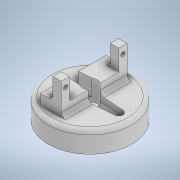
# Autodesk Inventor part: Part1
Saved by Autodesk Inventor 2020.2 (Build 242310000, 310)
## iProperties
Created: 2026-04-23
Part Number: Part1
Material: Generic
Document SubType Name: Modeling
Designer: explorer
Density: 1 g/cm^3
Appearance: Default
Author: explorer
Autodesk Inventor part; units mm, degrees
ref_plane "YZ Plane" through (0, 0, 0) normal (1, 0, 0) x (0, 1, 0)
ref_plane "XZ Plane" through (0, 0, 0) normal (0, 1, 0) x (-1, 0, 0)
ref_plane "XY Plane" through (0, 0, 0) normal (0, 0, 1) x (1, 0, 0)
sketch "Sketch1" plane through (0, 0, 0) normal (0, 1, 0) x (-1, 0, 0)
  circle A0 centre (0, 0) radius 20
  circle A1 centre (0, 0) radius 3.5
  dimension "d10" = 40
  dimension "d115" = 7
  constraints: 2 centre point, 2 coincident
  measures "d10" diameter of A0
  measures "d115" diameter of A1
extrude "Extrusion1" add sketch "Sketch1" along normal blind 10
sketch "Sketch3" plane through (0, 0, 0) normal (0, -1, 0) x (1, 0, 0)
  circle A0 centre (0, 0) radius 15
  dimension "d16" = 30
  constraints: 1 centre point, 1 coincident
  measures "d16" diameter of A0
extrude "Extrusion3" cut sketch "Sketch3" against normal blind 5
sketch "Sketch4" plane through (0, 10, 0) normal (0, 1, 0) x (1, 0, 0)
  circle A0 centre (-15.75, 0) radius 2 construction
  line L0 (0, 0) -> (-15.75, 0) construction
  arc A1 (-13.75, 2) -> (-13.75, -2) centre (-13.75, 0) ccw
  line L1 (-13.75, 0) -> (-13.75, 2) construction
  line L2 (-13.75, 0) -> (-11.75, 0) construction
  line L3 (-13.75, 0) -> (-13.75, -2) construction
  circle A2 centre (0, 0) radius 3.5 construction
  circle A3 centre (0, 0) radius 3 construction
  line L4 (0, 28) -> (0, -28) construction
  line L5 (-28, 0) -> (28, 0) construction
  line L6 (-13.75, 2) -> (0, 3)
  line L7 (-13.75, -2) -> (0, -3)
  arc A4 (13.75, -2) -> (13.75, 2) centre (13.75, 0) ccw
  line L8 (13.75, 2) -> (0, 3)
  line L9 (13.75, -2) -> (0, -3)
  dimension "d11" = 4
  dimension "d70" = 2
  dimension "d71" = 90
  dimension "d72" = 180
  dimension "d76" = 7
  dimension "d77" = 6
  dimension "d78" = 27.5
  constraints: 16 end point, 6 point on circle, 4 centre point, 3 coincident, 3 point on line, 3 symmetric about line, 2 horizontal, 1 horizontal alignment, 1 perpendicular, 3 other
  measures "d70" radius of A1
  measures "d71" angle of L2 L1
  measures "d72" angle of L1 L3
  measures "d76" diameter of A2
  measures "d77" diameter of A3
  measures "d78" distance of A4.centre L1.start
extrude "Extrusion4" cut sketch "Sketch4" against normal blind 2.75
sketch "Sketch16" plane through (0, 10, 0) normal (0, 1, 0) x (1, 0, 0)
  line L0 (-2, 15.75) -> (2, 15.75)
  line L1 (2, 15.75) -> (2, 11.75)
  line L2 (2, 11.75) -> (-2, 11.75)
  line L3 (-2, 11.75) -> (-2, 15.75)
  line L4 (0, 13.75) -> (0, 0) construction
  line L5 (-2, 15.75) -> (2, 11.75) construction
  line L6 (-28, 0) -> (28, 0) projected
  line L7 (0, 28) -> (0, -28) projected
  line L8 (-2, -15.75) -> (2, -15.75)
  line L9 (2, -15.75) -> (2, -11.75)
  line L10 (2, -11.75) -> (-2, -11.75)
  line L11 (-2, -11.75) -> (-2, -15.75)
  dimension "d117" = 4
  dimension "d118" = 13.75
  dimension "d121" = 23.5
  constraints: 20 end point, 4 symmetric about line, 2 parallel, 2 perpendicular, 1 horizontal, 1 midpoint, 1 vertical
  measures "d117" distance of L0.end L1.end
  measures "d118" distance of L4.start L4.end
  measures "d121" distance between parallel lines of L10 L2
extrude "Extrusion12" add sketch "Sketch16" along normal blind 15
sketch "Sketch17" plane through (2, 10, -11.75) normal (1, 0, 0) x (0, 0, -1)
  line L0 (0, 0) -> (0, 15) projected
  line L1 (4, 0) -> (4, 15) projected
  line L2 (0, 0) -> (4, 0) construction
  line L3 (4, 0) -> (0, 0) construction
  line L4 (2, 0) -> (2, 11.5) construction
  line L5 (-11.75, 0) -> (-11.75, 14.3038) construction
  circle A0 centre (2, 11.5) radius 1
  circle A1 centre (-25.5, 11.5) radius 1
  point P0 (-11.75, -10)
  dimension "d122" = 2
  dimension "d123" = 11.5
  constraints: 6 end point, 2 centre point, 2 vertical, 1 coincident, 1 midpoint, 1 perpendicular, 1 symmetric about line, 1 other
  measures "d122" diameter of A0
  measures "d123" distance of L4.start L4.end
extrude "Extrusion13" cut sketch "Sketch17" against normal up to surface (4 mm away)
sketch "Sketch18" plane through (2, 10, -11.75) normal (1, 0, 0) x (0, 0, -1)
  line L0 (-27.5, 0) -> (-27.5, 15) projected
  line L1 (4, 0) -> (4, 15) projected
  line L2 (-27.5, 0) -> (4, 0)
  line L3 (4, 0) -> (4, 5)
  line L4 (4, 5) -> (-27.5, 5)
  line L5 (-27.5, 5) -> (-27.5, 0)
  point P0 (-11.75, -10)
  point P1 (-27.5, 5)
  dimension "d126" = 5
  constraints: 8 end point, 2 parallel, 1 horizontal, 1 perpendicular, 1 point on line
  measures "d126" distance of L2.end L3.end
extrude "Extrusion14" add sketch "Sketch18" against normal blind 10
sketch "Sketch19" plane through (2, 15, 11.75) normal (0, 1, 0) x (1, 0, 0)
  circle A0 centre (-2, 11.75) radius 3.5
  circle A1 centre (-2, 11.75) radius 3.5 projected
  arc A2 (-15.75, 13.75) -> (-15.75, 9.75) centre (-15.75, 11.75) ccw projected
  line L0 (-2, 11.75) -> (-15.75, 11.75)
  circle A3 centre (-15.75, 11.75) radius 2
  line L1 (-15.75, 13.75) -> (-4.0281, 14.6025) projected
  line L2 (-15.75, 13.75) -> (-4.0281, 14.6025)
  line L3 (-4.0281, 8.8975) -> (-15.75, 9.75) projected
  line L4 (-4.0281, 14.6025) -> (-4.0281, 8.8975)
  line L5 (-4.0281, 8.8975) -> (-15.75, 9.75)
  dimension "d129" = 7
  constraints: 8 end point, 2 centre point, 2 coincident, 1 collinear, 1 concentric, 1 horizontal, 1 vertical
  measures "d129" diameter of A0
extrude "Extrusion15" cut sketch "Sketch19" against normal up to surface (7.75 mm away)
fillet "Fillet8" radius 2 1 edges at (20, 10, 0)
fillet "Fillet10" radius 2 4 edges at (2, 10, 9.3111) (2, 10, -9.3111) (-2, 15, 13.75) (-2, 15, -13.75)
body "Solid1"
